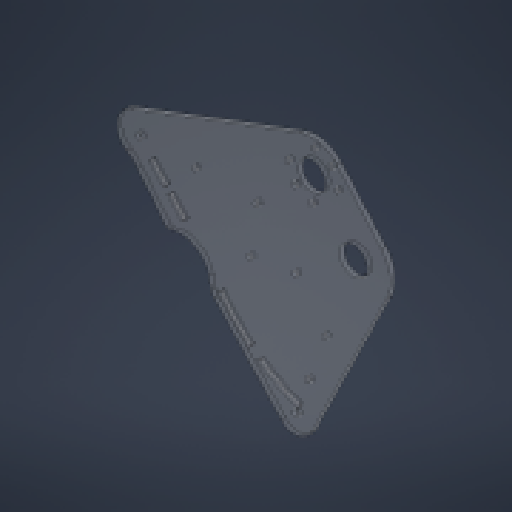
# Autodesk Inventor part: 4Bar_Input Side
Saved by Autodesk Inventor 2026 (Build 300175000, 175)
## iProperties
Created: 2026-01-17
Part Number: 4Bar_Input Side
Material: Polycarbonate, Clear
Document SubType Name: Modeling
Designer: 110
Density: 1.2 g/cm^3
Appearance: Polycarbonate - Clear
Mass: 240.06 g
Surface Area: 914.063 cm^2
Volume: 200.05 cm^3
Author: 110
Autodesk Inventor part; units mm, degrees
ref_plane "YZ Plane" through (0, 0, 0) normal (1, 0, 0) x (0, 1, 0)
ref_plane "XZ Plane" through (0, 0, 0) normal (0, 1, 0) x (-1, 0, 0)
ref_plane "XY Plane" through (0, 0, 0) normal (0, 0, 1) x (1, 0, 0)
sketch "Sketch1" plane through (0, 0, 0) normal (0, 0, 1) x (1, 0, 0)
  arc A0 (-7.9109, 20.947) -> (-12.5617, -18.5355) centre (0, 0) ccw
  circle A1 centre (222.25, 0) radius 38.1 construction
  arc A2 (256.45, -16.7919) -> (250.9516, 25.0564) centre (222.25, 0) ccw
  arc A3 (147.4862, -180.0475) -> (178.5388, -175.4733) centre (161.4388, -167.0773) ccw
  line L0 (0, 0) -> (203.2, 0) construction
  line L1 (222.25, 0) -> (161.4388, -167.0773) construction
  line L2 (0, 149.2071) -> (0, -244.4474) construction
  line L3 (-102.8675, 0) -> (329.7763, 0) construction
  line L4 (0, 0) -> (222.25, 0) construction
  circle A4 centre (187.8917, -94.3987) radius 75.057 construction
  circle A5 centre (222.25, 0) radius 25.4 construction
  circle A6 centre (179.1089, 54.2451) radius 25.4 construction
  arc A7 (205.4187, 77.2135) -> (166.7696, 86.9176) centre (179.1089, 54.2451) ccw
  line L5 (205.4187, 77.2135) -> (250.9516, 25.0564)
  line L6 (166.7696, 86.9176) -> (-7.9109, 20.947)
  line L7 (222.25, 0) -> (179.1089, 54.2451) construction
  circle A8 centre (222.25, 0) radius 45.72 construction
  arc A9 (72.7614, -88.5895) -> (32.1142, -67.3414) centre (43.3613, -95.3285) ccw
  line L8 (43.3613, -95.3285) -> (-19.8796, -15.8102) construction
  line L9 (-19.8796, -15.8102) -> (0, 0) construction
  line L10 (28.4453, -66.3716) -> (-1.3022, -28.9676)
  arc A10 (28.4453, -66.3716) -> (32.1142, -67.3414) centre (30.9303, -64.3953) ccw
  arc A11 (-1.3022, -28.9676) -> (-12.5617, -18.5355) centre (-41.0613, -60.588) ccw
  line L11 (72.7614, -88.5895) -> (75.3699, -99.9695)
  line L12 (256.45, -16.7919) -> (178.5388, -175.4733)
  arc A12 (81.8064, -98.3397) -> (163.6106, -161.1103) centre (222.25, 0) ccw
  line L13 (222.25, 0) -> (81.8064, -98.3397) construction
  line L14 (222.25, 0) -> (163.6106, -161.1103) construction
  line L15 (81.8064, -98.3397) -> (84.4072, -96.5186)
  arc A13 (84.4072, -96.5186) -> (164.6966, -158.1268) centre (222.25, 0) ccw
  arc A14 (115.2139, -129.8451) -> (124.5322, -136.9953) centre (222.25, 0) ccw
  line L16 (115.2139, -129.8451) -> (113.1944, -132.295)
  line L17 (124.5322, -136.9953) -> (122.6885, -139.5801)
  line L18 (12.958, -13.9669) -> (46.9467, -51.7215)
  line L19 (25.3128, -32.7489) -> (27.8281, -30.4845)
  line L20 (32.0767, -35.2038) -> (29.5614, -37.4682)
  line L21 (27.8281, -30.4845) -> (32.0767, -35.2038)
  line L22 (10.5984, -16.0912) -> (44.5871, -53.8458)
  line L23 (44.5871, -53.8458) -> (46.9467, -51.7215)
  line L24 (12.958, -13.9669) -> (10.5984, -16.0912)
  line L25 (160.1656, -159.8564) -> (167.0557, -162.3642) construction
  line L26 (167.0557, -162.3642) -> (168.329, -169.5852) construction
  line L27 (168.329, -169.5852) -> (162.7121, -174.2983) construction
  line L28 (162.7121, -174.2983) -> (155.8219, -171.7905) construction
  line L29 (155.8219, -171.7905) -> (154.5487, -164.5695) construction
  line L30 (154.5487, -164.5695) -> (160.1656, -159.8564) construction
  line L31 (161.4388, -167.0773) -> (163.6106, -161.1103) construction
  line L32 (163.6106, -161.1103) -> (164.6966, -158.1268)
  line L33 (147.4862, -180.0475) -> (78.4471, -105.7788)
  arc A15 (75.3699, -99.9695) -> (78.4471, -105.7788) centre (87.7488, -97.132) ccw
  point P0 (193.7916, 35.7832)
  point P1 (-2.1435, -27.9096)
  point P2 (119.8107, -133.5015)
  point P3 (29.9524, -32.8442)
  point P4 (25.4684, -32.6088)
  point P5 (29.717, -37.3281)
  dimension "d30" = 76.2
  dimension "d110" = 91.44
  dimension "d31" = 44.7822
  dimension "d34" = 177.8
  dimension "d39" = 19.05
  dimension "d80" = 22.3911
  dimension "d86" = 222.25
  dimension "d87" = 0
  dimension "d101" = 70
  dimension "d102" = 150.114
  dimension "d103" = 50.8
  dimension "d107" = 69.3086
  dimension "d108" = 59.0923
  dimension "d109" = 34.925
  dimension "d139" = 60.325
  dimension "d140" = 25.4
  dimension "d141" = 101.6
  dimension "d143" = 3.175
  dimension "d176" = 6.35
  dimension "d180" = 171.45
  dimension "d181" = 35
  dimension "d192" = 50.8
  dimension "d194" = 4
  dimension "d195" = 6.35
  dimension "d198" = 50.8
  dimension "d200" = 3.175
  dimension "d201" = 19.05
  dimension "d202" = 3.5
  dimension "d203" = 172.72
  dimension "d204" = 12.7
  dimension "d205" = 168.275
  dimension "d206" = 177.8
  dimension "d216" = 12.7
  dimension "d217" = 150
  dimension "d218" = 101.6
  constraints: 64 end point, 30 point on circle, 14 centre point, 14 tangent, 11 coincident, 9 point on line, 5 perpendicular, 3 collinear, 3 line through centre, 3 midpoint, 2 parallel, 1 concentric, 1 equal radius, 21 other
  measures "d31" diameter of A0
  measures "d34" distance of L1.start L1.end
  measures "d39" radius of A3
  measures "d80" radius of A0
  measures "d86" distance of L0.start L1.start
  measures "d87" distance between parallel lines of L4 L0
  measures "d101" angle of L0 L1
  measures "d102" diameter of A4
  measures "d103" diameter of A5
  measures "d107" distance of point (179.109, 54.245) L1.start
  measures "d108" distance from line of point (179.109, 54.245) L1
  measures "d109" radius of A7
  measures "d139" diameter of A9
  measures "d140" distance of L8.end L0.start
  measures "d141" distance of L8.start L8.end
  measures "d143" radius of A10
  measures "d176" distance between parallel lines of L8 L10
  measures "d180" radius of A12
  measures "d181" angle of L13 L14
  measures "d192" radius of A11
  measures "d194" angle of L16 L17
  measures "d195" distance between parallel lines of L19 L20
  measures "d198" distance of L18.start L18.end
  measures "d200" distance of L22.end L18.end
  measures "d201" distance from line of A0.centre L24
  measures "d202" angle of L8 L22
  measures "d203" distance of point (179.109, 54.245) point (29.952, -32.844)
  measures "d204" distance between parallel lines of L28 L25
  measures "d205" radius of A13
  measures "d206" distance of point (222.25, 0) A3.centre
  measures "d216" radius of A15
  measures "d217" angle of L33 L11
  measures "d218" distance of A3.centre A15.centre
extrude "Extrusion1" add sketch "Sketch1" along normal blind 4.7625 contours L6 A7 L5 A2 L12 A3 L33 A15 L11 A9 A10 L10 A11 A0 | L16 A13 L17 A12 | L18 L20 L22 L19
sketch "Sketch2" plane through (0, 0, 4.7625) normal (0, 0, 1) x (1, 0, 0)
  arc A0 (147.4862, -180.0475) -> (178.5388, -175.4733) centre (161.4388, -167.0773) ccw projected
  arc A1 (-7.9109, 20.947) -> (-12.5617, -18.5355) centre (0, 0) ccw projected
  line L0 (178.5388, -175.4733) -> (256.45, -16.7919) projected
  arc A2 (256.45, -16.7919) -> (250.9516, 25.0564) centre (222.25, 0) ccw projected
  line L1 (166.7696, 86.9176) -> (-7.9109, 20.947) projected
  line L2 (250.9516, 25.0564) -> (205.4187, 77.2135) projected
  arc A3 (205.4187, 77.2135) -> (166.7696, 86.9176) centre (179.1089, 54.2451) ccw projected
  line L3 (-1.3022, -28.9676) -> (28.4453, -66.3716) projected
  arc A4 (72.7614, -88.5895) -> (32.1142, -67.3414) centre (43.3613, -95.3285) ccw projected
  arc A5 (-1.3022, -28.9676) -> (-12.5617, -18.5355) centre (-41.0613, -60.588) ccw projected
  arc A6 (28.4453, -66.3716) -> (32.1142, -67.3414) centre (30.9303, -64.3953) ccw projected
  line L4 (72.7614, -88.5895) -> (75.3699, -99.9695) projected
  arc A7 (75.3699, -99.9695) -> (78.4471, -105.7788) centre (87.7488, -97.132) ccw projected
  line L5 (78.4471, -105.7788) -> (147.4862, -180.0475) projected
  constraints: 1 coincident
hole "Structure Holes" at (0, 0, 4.7625) direction (0, 0, -1) diameter 6.35 end through all
sketch "Sketch4" plane through (0, 0, 4.7625) normal (0, 0, 1) x (1, 0, 0)
  arc A0 (147.4862, -180.0475) -> (178.5388, -175.4733) centre (161.4388, -167.0773) ccw projected
  arc A1 (-7.9109, 20.947) -> (-12.5617, -18.5355) centre (0, 0) ccw projected
  line L0 (178.5388, -175.4733) -> (256.45, -16.7919) projected
  arc A2 (256.45, -16.7919) -> (250.9516, 25.0564) centre (222.25, 0) ccw projected
  line L1 (0, 0) -> (114.3, -50.8) construction
  line L2 (166.7696, 86.9176) -> (-7.9109, 20.947) projected
  line L3 (250.9516, 25.0564) -> (205.4187, 77.2135) projected
  arc A3 (205.4187, 77.2135) -> (166.7696, 86.9176) centre (179.1089, 54.2451) ccw projected
  line L4 (179.1089, 54.2451) -> (271.2167, -45.4479) construction
  line L5 (-1.3022, -28.9676) -> (28.4453, -66.3716) projected
  arc A4 (72.7614, -88.5895) -> (32.1142, -67.3414) centre (43.3613, -95.3285) ccw projected
  arc A5 (-1.3022, -28.9676) -> (-12.5617, -18.5355) centre (-41.0613, -60.588) ccw projected
  arc A6 (28.4453, -66.3716) -> (32.1142, -67.3414) centre (30.9303, -64.3953) ccw projected
  line L6 (72.7614, -88.5895) -> (75.3699, -99.9695) projected
  arc A7 (75.3699, -99.9695) -> (78.4471, -105.7788) centre (87.7488, -97.132) ccw projected
  line L7 (78.4471, -105.7788) -> (147.4862, -180.0475) projected
  point P0 (153.7287, 55.2488)
  point P1 (160.4527, 37.0083)
  point P2 (178.1052, 28.8649)
  point P3 (196.3456, 35.5888)
  point P4 (204.489, 53.2413)
  point P5 (197.7651, 71.4818)
  point P6 (180.1126, 79.6252)
  point P7 (161.8721, 72.9013)
  dimension "d83" = 114.3
  dimension "d84" = 50.8
  dimension "d132" = 25.4
  dimension "d135" = 360
  constraints: 4 end point, 3 coincident, 1 point on line, 9 other
  measures "d83" horizontal distance of L1.start L1.end
  measures "d84" vertical distance of L1.start L1.end
  measures "d132" distance of L4.start point (153.729, 55.249)
hole "BearingHole" at (222.25, 0, 4.7625) at (179.1089, 54.2451, 4.7625) direction (0, 0, -1) diameter 28.575 end through all
hole "Hole4" at (114.3, -50.8, 4.7625) direction (0, 0, -1) diameter 5.1054 end through all clearance for "Socket Head Cap Screw" size "#10" standard "Ansi Unified Screw Threads"
sketch "Sketch3" plane through (0, 0, 0) normal (0, 0, -1) x (-1, 0, 0)
  line L0 (0, 0) -> (-222.25, 0) construction
  line L1 (-222.25, 0) -> (-159.267, -173.0444) construction
  line L2 (-84.8185, 0) -> (-175.2456, -129.1434) construction
  line L3 (-130.032, -64.5717) -> (-161.2417, -42.7184) construction
  point P0 (-184.15, 0)
  point P1 (-120.65, 0)
  point P2 (-57.15, 0)
  point P3 (-209.219, -35.8023)
  point P4 (-191.8444, -83.5387)
  point P5 (-174.4698, -131.2751)
  dimension "d10" = 137.4315
  dimension "d11" = 137.4315
  dimension "d12" = 38.1
  dimension "d43" = 38.1
  dimension "d46" = 63.5
  dimension "d51" = 38.1
  dimension "d54" = 50.8
  constraints: 8 end point, 4 point on line, 2 coincident, 1 horizontal, 1 midpoint, 1 perpendicular, 5 other
  measures "d10" distance of L0.end L2.end
  measures "d11" distance of L0.end L2.start
  measures "d12" distance of L3.start L3.end
  measures "d43" distance of point (-184.15, 0) L0.end
  measures "d46" distance of point (-184.15, 0) point (-120.65, 0)
  measures "d51" distance of point (-209.219, -35.802) L0.end
  measures "d54" distance of point (-209.219, -35.802) point (-191.844, -83.539)
ref_plane "Inner Pitch Plane" through (0, 0, 0) normal (1, 0, 0) x (0, 1, 0)
hole "Hole6" at (180.1126, 79.6252, 4.7625) at (197.7651, 71.4818, 4.7625) at (204.489, 53.2413, 4.7625) at (178.1052, 28.8649, 4.7625) at (160.4527, 37.0083, 4.7625) at (153.7287, 55.2488, 4.7625) direction (0, 0, -1) diameter 4.9784 end through all clearance for "Flat Head Machine Screw (82)" size "#10" standard "Ansi Unified Screw Threads"
hole "Hole8" at (161.2417, -42.7184, 0) at (0, 0, 0) at (222.25, 0, 0) at (120.65, 0, 0) at (57.15, 0, 0) at (191.8444, -83.5387, 0) at (174.4698, -131.2751, 0) direction (0, 0, 1) diameter 5.1054 end through all clearance for "Flat Head Machine Screw (82)" size "#10" standard "Ansi Unified Screw Threads"
hole "Hole9" at (161.4388, -167.0773, 0) direction (0, 0, 1) diameter 6.5278 end through all clearance for "Flat Head Machine Screw (82)" size "1/4" standard "Ansi Unified Screw Threads"
equation "\"d10\" = d11"
equation "\"d51\" = d43"
body "Solid1"
